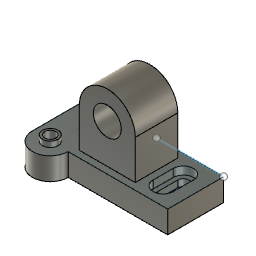
drawing_22 (Autodesk Fusion 360 design; units mm, degrees)
Autodesk Fusion 360 part; units mm, degrees
sketch "Sketch1" plane through (0, 0, 0) normal (0, 0, 1) x (1, 0, 0)
  line L0 (28.5, 25) -> (-60.5, 25)
  line L1 (-60.5, -25) -> (28.5, -25)
  line L2 (60.5, 25) -> (-60.5, -25) construction
  line L3 (-60.5, 25) -> (60.5, -25) construction
  line L4 (-92.5, 25) -> (-92.5, -25)
  arc A0 (-92.5, -25) -> (-60.5, -25) centre (-76.5, -25) ccw
  arc A1 (-60.5, 25) -> (-92.5, 25) centre (-76.5, 25) ccw
  line L5 (-76.5, 25) -> (-76.5, -25) construction
  line L6 (28.5, 25) -> (28.5, -25)
  line L7 (28.5, 25) -> (28.5, -25)
  line L8 (-60.5, 25) -> (28.5, 25)
  dimension "d1" = 121
  dimension "d2" = 50
  dimension "d3" = 16
  dimension "d4" = 32
  dimension "d5" = 121
  constraint horizontal L0
  constraint parallel L0 L1
  constraint coincident L2 origin
  constraint coincident L3 origin
  constraint tangent L4 A0
  constraint tangent L4 A1
  constraint perpendicular L1 L6
  measures "d1" distance of L1.start L3.end
  measures "d2" distance of L0.end L1.start
  measures "d3" distance of L0.end A1.centre
  measures "d4" diameter of A0
  measures "d5" distance of L4.start L0.start
extrude "Extrude1" add sketch "Sketch1" along normal blind 20
sketch "Sketch2" plane through (0, 0, 20) normal (0, 0, 1) x (-1, 0, 0)
  line L0 (92.5, -25) -> (92.5, 25)
  arc A0 (92.5, 25) -> (60.5, 25) centre (76.5, 25) ccw
  line L1 (60.5, 25) -> (-28.5, 25)
  line L2 (-28.5, 25) -> (-28.5, -25)
  line L3 (-28.5, -25) -> (60.5, -25)
  arc A1 (60.5, -25) -> (92.5, -25) centre (76.5, -25) ccw
  circle A2 centre (76.5, -25) radius 7
  circle A3 centre (76.5, 25) radius 7
  circle A4 centre (76.5, -25) radius 5
  circle A5 centre (76.5, 25) radius 5
  dimension "d8" = 14
  dimension "d9" = 14
  dimension "d10" = 10
  dimension "d11" = 10
  constraint concentric A1 A2
  constraint concentric A0 A3
  constraint concentric A2 A4
  constraint concentric A3 A5
  measures "d8" diameter of A2
  measures "d9" diameter of A3
  measures "d10" diameter of A4
  measures "d11" diameter of A5
extrude "Extrude2" cut sketch "Sketch2" against normal blind 45 contours A4 | A5
sketch "Sketch3" plane through (0, 0, 20) normal (0, 0, 1) x (-1, 0, 0)
  circle A0 centre (76.5, 25) radius 5
  circle A1 centre (76.5, -25) radius 5
  line L0 (92.5, -25) -> (92.5, 25)
  arc A2 (92.5, 25) -> (60.5, 25) centre (76.5, 25) ccw
  line L1 (60.5, 25) -> (-28.5, 25)
  line L2 (-28.5, 25) -> (-28.5, -25)
  line L3 (-28.5, -25) -> (60.5, -25)
  arc A3 (60.5, -25) -> (92.5, -25) centre (76.5, -25) ccw
  circle A4 centre (76.5, -25) radius 7
  circle A5 centre (76.5, 25) radius 7
  dimension "d14" = 14
  dimension "d15" = 14
  constraint concentric A1 A4
  constraint concentric A0 A5
  measures "d14" diameter of A4
  measures "d15" diameter of A5
extrude "Extrude3" add sketch "Sketch3" along normal blind 5 contours A4 | A5
sketch "Sketch4" plane through (0, 0, 0) normal (0, 0, -1) x (1, 0, 0)
  circle A0 centre (-76.5, 25) radius 5
  circle A1 centre (-76.5, -25) radius 5
  line L0 (-92.5, 25) -> (-92.5, -25)
  arc A2 (-92.5, -25) -> (-60.5, -25) centre (-76.5, -25) ccw
  line L1 (-60.5, -25) -> (28.5, -25)
  line L2 (28.5, -25) -> (28.5, 25)
  line L3 (28.5, 25) -> (-60.5, 25)
  arc A3 (-60.5, 25) -> (-92.5, 25) centre (-76.5, 25) ccw
  line L4 (-86.5, 25) -> (-86.5, -25)
  arc A4 (-86.5, -25) -> (-66.5, -25) centre (-76.5, -25) ccw
  arc A5 (-66.5, 25) -> (-86.5, 25) centre (-76.5, 25) ccw
  line L5 (-76.5, 25) -> (-76.5, -25) construction
  line L6 (-30, 25) -> (-30, 19) construction
  line L7 (28.5, 0) -> (22.5, 0) construction
  line L8 (22.5, 19) -> (22.5, 0)
  line L9 (22.5, 19) -> (-66.5, 19)
  line L10 (22.5, 0) -> (22.5, -19)
  line L11 (22.5, -19) -> (-66.5, -19)
  line L12 (-66.5, -25) -> (-66.5, -19)
  line L13 (-66.5, 19) -> (-66.5, 25)
  dimension "d18" = 20
  dimension "d19" = 6
  dimension "d20" = 6
  dimension "d21" = 19
  constraint tangent L4 A4
  constraint tangent A4 L12
  constraint parallel L4 L12
  constraint tangent A5 L12
  constraint tangent L4 A5
  constraint coincident A1.centre A2.centre
  constraint vertical L5
  constraint coincident A0.centre A3.centre
  constraint coincident L3 L6.start
  constraint perpendicular L3 L6
  constraint midpoint L2 L7.start
  constraint perpendicular L2 L7
  constraint perpendicular L7 L8
  constraint coincident L9.end L12
  constraint perpendicular L9 L12
  constraint perpendicular L9 L10
  constraint perpendicular L11 L12
  constraint collinear L12 L13
  measures "d18" diameter of A4
  measures "d19" distance of L6.start L6.end
  measures "d20" distance of L7.start L7.end
  measures "d21" distance of L7.end L10.end
extrude "Extrude4" cut sketch "Sketch4" against normal blind 7 contours L4 A4 A5 L8 L9 L10 L11 L12 L13
sketch "Sketch5" plane through (0, 0, 20) normal (0, 0, 1) x (-1, 0, 0)
  circle A0 centre (76.5, 25) radius 7
  circle A1 centre (76.5, -25) radius 7
  line L0 (92.5, -25) -> (92.5, 25)
  arc A2 (92.5, 25) -> (60.5, 25) centre (76.5, 25) ccw
  line L1 (60.5, 25) -> (-28.5, 25)
  line L2 (-28.5, 25) -> (-28.5, -25)
  line L3 (-28.5, -25) -> (60.5, -25)
  arc A3 (60.5, -25) -> (92.5, -25) centre (76.5, -25) ccw
  line L4 (-28.5, 0) -> (-28.5, -9)
  line L5 (-28.5, 0) -> (-28.5, 9)
  line L6 (-28.5, -25) -> (-8.5, -25)
  line L7 (-8.5, -9) -> (-8.5, 9)
  line L8 (0.5, -9) -> (0.5, 9)
  arc A4 (0.5, 9) -> (-17.5, 9) centre (-8.5, 9) ccw
  line L9 (-17.5, 9) -> (-17.5, -9)
  arc A5 (-17.5, -9) -> (0.5, -9) centre (-8.5, -9) ccw
  line L10 (-8.5, -9) -> (-8.5, 9) construction
  line L11 (-3.5, -9) -> (-3.5, 9)
  arc A6 (-3.5, 9) -> (-13.5, 9) centre (-8.5, 9) ccw
  line L12 (-13.5, 9) -> (-13.5, -9)
  arc A7 (-13.5, -9) -> (-3.5, -9) centre (-8.5, -9) ccw
  line L13 (-8.5, -9) -> (-8.5, 9) construction
  dimension "d24" = 9
  dimension "d25" = 9
  dimension "d26" = 20
  dimension "d27" = 18
  dimension "d28" = 10
  constraint midpoint L2 L4.start
  constraint perpendicular L3 L4
  constraint perpendicular L3 L5
  constraint coincident L2.end L3.start
  constraint perpendicular L2 L6
  constraint perpendicular L6 L7
  constraint tangent L8 A4
  constraint tangent A4 L9
  constraint parallel L8 L9
  constraint tangent L9 A5
  constraint tangent L8 A5
  constraint coincident L7.end A4.centre
  constraint perpendicular L3 L10
  constraint coincident L7.start A5.centre
  constraint tangent L11 A6
  constraint tangent A6 L12
  constraint parallel L11 L12
  constraint tangent L12 A7
  constraint tangent L11 A7
  constraint parallel L7 L13
  measures "d24" distance of L4.start L4.end
  measures "d25" distance of L4.start L5.end
  measures "d26" distance of L2.end L6.end
  measures "d27" diameter of A4
  measures "d28" diameter of A6
extrude "Extrude5" cut sketch "Sketch5" against normal blind 7 contours L8 A4 L9 A5
extrude "Extrude6" cut 1 faces at (10.1667, -3, 20) along direction (0, 0, -1) blind 55
sketch "Sketch6" plane through (0, 0, 20) normal (0, 0, 1) x (-1, 0, 0)
  line L0 (92.5, -25) -> (92.5, 25)
  arc A0 (92.5, 25) -> (60.5, 25) centre (76.5, 25) ccw
  line L1 (60.5, 25) -> (-28.5, 25)
  line L2 (-28.5, 25) -> (-28.5, -25)
  line L3 (-28.5, -25) -> (60.5, -25)
  arc A1 (60.5, -25) -> (92.5, -25) centre (76.5, -25) ccw
  circle A2 centre (76.5, -25) radius 7
  circle A3 centre (76.5, 25) radius 7
  line L4 (0.5, 9) -> (0.5, -9)
  arc A4 (-17.5, -9) -> (0.5, -9) centre (-8.5, -9) ccw
  line L5 (-17.5, -9) -> (-17.5, 9)
  arc A5 (0.5, 9) -> (-17.5, 9) centre (-8.5, 9) ccw
sketch "Sketch7" plane through (0, 0, 20) normal (0, 0, 1) x (-1, 0, 0)
  line L0 (-28.5, -25) -> (31.5, -25)
  dimension "d33" = 60
  constraint horizontal L0
  measures "d33" distance of L0.start L0.end
sketch "Sketch8" plane through (0, 0, 20) normal (0, 0, 1) x (-1, 0, 0)
  line L0 (31.5, -25) -> (31.5, 0)
  arc A0 (-13.5, -9) -> (-3.5, -9) centre (-8.5, -9) ccw
  line L1 (-3.5, -9) -> (-3.5, 9)
  arc A1 (-3.5, 9) -> (-13.5, 9) centre (-8.5, 9) ccw
  line L2 (-13.5, 9) -> (-13.5, -9)
  circle A2 centre (76.5, 25) radius 5
  circle A3 centre (76.5, -25) radius 5
  line L3 (-22.5, 19) -> (66.5, 19)
  line L4 (66.5, 19) -> (66.5, 25)
  arc A4 (86.5, 25) -> (66.5, 25) centre (76.5, 25) ccw
  line L5 (86.5, 25) -> (86.5, -25)
  arc A5 (66.5, -25) -> (86.5, -25) centre (76.5, -25) ccw
  line L6 (66.5, -25) -> (66.5, -19)
  line L7 (66.5, -19) -> (-22.5, -19)
  line L8 (-22.5, -19) -> (-22.5, 19)
  line L9 (31.5, -19) -> (56.5, -19)
  line L10 (31.5, 19) -> (6.5, 19)
  line L11 (6.5, 19) -> (56.5, 19)
  line L12 (56.5, 19) -> (56.5, -19)
  line L13 (56.5, -19) -> (6.5, -19)
  line L14 (6.5, -19) -> (6.5, 19)
  dimension "d34" = 25
  dimension "d35" = 25
  constraint vertical L0
  constraint coincident L0 L9.start
  constraint coincident L7 L9.start
  constraint perpendicular L0 L9
  constraint coincident L3 L10.start
  constraint perpendicular L0 L10
  constraint horizontal L11
  constraint vertical L12
  constraint horizontal L13
  constraint vertical L14
  measures "d34" distance of L9.start L9.end
  measures "d35" distance of L10.start L10.end
extrude "Extrude7" add sketch "Sketch8" along normal blind 35 contours L3 L7 L9 L10 L11 L12 L13 L14
sketch "Sketch9" plane through (0, -19, 0) normal (0, -1, 0) x (1, 0, 0)
  line L0 (-56.5, 20) -> (-6.5, 20)
  line L1 (-6.5, 20) -> (-6.5, 55)
  line L2 (-6.5, 55) -> (-56.5, 55)
  line L3 (-56.5, 55) -> (-56.5, 20)
  circle A0 centre (-31.5, 55) radius 25
  dimension "d38" = 50
  constraint midpoint L2 A0.centre
  measures "d38" diameter of A0
extrude "Extrude8" add sketch "Sketch9" against normal blind 38 contours L2 A0 picked at (-35.1673, 71.0673)
sketch "Sketch10" plane through (0, -19, 0) normal (0, -1, 0) x (1, 0, 0)
  line L0 (-56.5, 20) -> (-6.5, 20)
  line L1 (-6.5, 20) -> (-6.5, 55)
  arc A0 (-6.5, 55) -> (-56.5, 55) centre (-31.5, 55) ccw
  line L2 (-56.5, 55) -> (-56.5, 20)
  circle A1 centre (-31.5, 55) radius 12.5
  dimension "d41" = 25
  constraint concentric A0 A1
  measures "d41" diameter of A1
extrude "Extrude9" cut sketch "Sketch10" against normal blind 70 contours A1
sketch "Sketch11" plane through (0, 0, 7) normal (0, 0, -1) x (1, 0, 0)
  arc A0 (3.5, -9) -> (13.5, -9) centre (8.5, -9) ccw
  line L0 (3.5, -9) -> (3.5, 9)
  arc A1 (13.5, 9) -> (3.5, 9) centre (8.5, 9) ccw
  line L1 (13.5, 9) -> (13.5, -9)
  circle A2 centre (-76.5, 25) radius 5
  circle A3 centre (-76.5, -25) radius 5
  line L2 (22.5, 19) -> (-66.5, 19)
  line L3 (-66.5, 19) -> (-66.5, 25)
  arc A4 (-66.5, 25) -> (-86.5, 25) centre (-76.5, 25) ccw
  line L4 (-86.5, 25) -> (-86.5, -25)
  arc A5 (-86.5, -25) -> (-66.5, -25) centre (-76.5, -25) ccw
  line L5 (-66.5, -25) -> (-66.5, -19)
  line L6 (-66.5, -19) -> (22.5, -19)
  line L7 (22.5, -19) -> (22.5, 19)
  line L8 (-66.5, 25) -> (-66.5, 19)
  line L9 (-66.5, 19) -> (22.5, 19)
  line L10 (22.5, 19) -> (22.5, -19)
  line L11 (22.5, -19) -> (-66.5, -19)
  line L12 (-66.5, -19) -> (-66.5, -25)
  arc A6 (-86.5, -25) -> (-66.5, -25) centre (-76.5, -25) ccw
  line L13 (-86.5, -25) -> (-86.5, 25)
  arc A7 (-66.5, 25) -> (-86.5, 25) centre (-76.5, 25) ccw
  line L14 (-92.5, 25) -> (-92.5, -25)
  arc A8 (-92.5, -25) -> (-60.5, -25) centre (-76.5, -25) ccw
  line L15 (-60.5, -25) -> (28.5, -25)
  line L16 (28.5, -25) -> (28.5, 25)
  line L17 (28.5, 25) -> (-60.5, 25)
  arc A9 (-60.5, 25) -> (-92.5, 25) centre (-76.5, 25) ccw
  line L18 (-92.5, 0) -> (-32, 0)
  circle A10 centre (-32, 0) radius 7
  dimension "d44" = 60.5
  dimension "d45" = 14
  constraint midpoint L14 L18.start
  constraint perpendicular L16 L18
  constraint coincident L18.end A10.centre
  measures "d44" distance of L18.start L18.end
  measures "d45" diameter of A10
extrude "Extrude10" cut sketch "Sketch11" against normal blind 8 contours A10
sketch "Sketch12" plane through (0, 0, 15) normal (0, 0, -1) x (1, 0, 0)
  circle A0 centre (-32, 0) radius 7
  circle A1 centre (-32, 0) radius 15
  dimension "d48" = 30
  constraint concentric A0 A1
  measures "d48" diameter of A1
extrude "Extrude11" cut sketch "Sketch12" against normal blind 15
extrude "Extrude12" cut 1 faces at (-31.572, 1.6695, 15) along direction (0, 0, 1) blind 15
equation "d2 = 0 mm + 50 mm"
equation "d44 = ( 121 / 2 ) * 1 mm"
